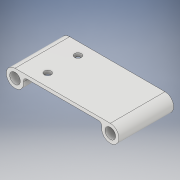
# Autodesk Inventor part: Turret Sensor Mount
Saved by Autodesk Inventor 2019.4 (Build 234330000, 330)
## iProperties
Created: 2020-01-25
Part Number: Turret Sensor Mount
Material: ABS Plastic
Document SubType Name: Modeling
Designer: admin
Density: 1.95534 g/cm^3
Appearance: Smooth - White
Mass: 200 g
Surface Area: 410.911 cm^2
Volume: 102.284 cm^3
Author: admin
Autodesk Inventor part; units mm, degrees
ref_plane "YZ Plane" through (0, 0, 0) normal (1, 0, 0) x (0, 1, 0)
ref_plane "XY Plane" through (0, 0, 0) normal (0, 0, 1) x (1, 0, 0)
sketch "Sketch1" plane through (0, 0, 0) normal (0, 0, 1) x (1, 0, 0)
  circle A0 centre (0, 0) radius 7.7
  circle A1 centre (0, 0) radius 12.7
  circle A2 centre (139.415, 0) radius 7.7
  circle A3 centre (139.415, 0) radius 12.7
  line L0 (0, 0) -> (139.415, 0) construction
  dimension "d0" = 15.4
  dimension "d1" = 15.4
  dimension "d2" = 139.415
  dimension "d3" = 5
  dimension "d4" = 5
  constraints: 4 centre point, 3 coincident, 2 end point, 1 horizontal
  measures "d0" diameter of A0
  measures "d1" diameter of A2
  measures "d2" distance of A2.centre A0.centre
  measures "d3" radial gap between concentric circles of A0 A1
  measures "d4" radial gap between concentric circles of A3 A2
extrude "Extrusion1" add sketch "Sketch1" along normal blind 80
ref_plane "Work Plane1" through (0, 12.7, 0) normal (0, 1, 0) x (-1, 0, 0)
sketch "Sketch2" plane through (0, 12.7, 0) normal (0, 1, 0) x (-1, 0, 0)
  line L0 (0, 0) -> (0, 80) projected
  line L1 (-139.415, 0) -> (-139.415, 80) projected
  line L2 (0, 80) -> (-139.415, 80)
  line L3 (-139.415, 80) -> (-139.415, 0)
  line L4 (-139.415, 0) -> (0, 0)
  line L5 (0, 0) -> (0, 80)
  line L6 (-30, 62.149) -> (-30, 17.851) construction
  line L7 (-35, 62.149) -> (-35, 17.851) construction
  line L8 (-25, 17.851) -> (-25, 62.149) construction
  arc A0 (-25, 62.149) -> (-35, 62.149) centre (-30, 62.149) ccw
  arc A1 (-35, 17.851) -> (-25, 17.851) centre (-30, 17.851) ccw
  circle A2 centre (-30, 62.149) radius 5
  circle A3 centre (-30, 17.851) radius 5
  line L9 (-30, 40) -> (-139.415, 40) construction
  dimension "d7" = 44.298
  dimension "d8" = 5
  dimension "d9" = 30
  constraints: 18 end point, 4 point on circle, 4 tangent, 3 parallel, 2 centre point, 2 coincident, 2 horizontal alignment, 2 midpoint, 2 perpendicular, 1 horizontal, 1 vertical, 4 other
  measures "d7" distance of L6.end L6.start
  measures "d8" radius of A1
  measures "d9" distance between parallel lines of L0 L6
extrude "Extrusion2" add sketch "Sketch2" against normal blind 5
fillet "Fillet1" radius 5 2 edges at (10.0995, 7.7, 40) (129.3155, 7.7, 40)
body "Solid1"
